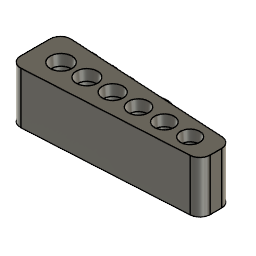
HoleDiaTest1.75mm_v3 (Autodesk Fusion 360 design; units mm, degrees)
Autodesk Fusion 360 part; units mm, degrees
sketch "Sketch1" plane through (0, 0, 0) normal (0, 0, 1) x (1, 0, 0)
  circle A0 centre (0, 0) radius 0.875
  circle A1 centre (2.5, 0) radius 0.85
  circle A2 centre (5, 0) radius 0.825
  circle A3 centre (-2.5, 0) radius 0.9
  circle A4 centre (-5, 0) radius 0.925
  circle A5 centre (-7.5, 0) radius 0.95
  line L0 (-7.5, 0) -> (5, 0) construction
  line L1 (5, 0) -> (7.5, 0) construction
  line L2 (-7.5, 0) -> (-10, 0) construction
  line L3 (-10, 2.5) -> (-10, -2.5)
  line L4 (7.5, 1.5) -> (7.5, -1.5)
  line L5 (7.5, 1.5) -> (-10, 2.5)
  line L6 (-10, -2.5) -> (7.5, -1.5)
  dimension "d1" = 1.75
  dimension "d2" = 1.7
  dimension "d3" = 1.65
  dimension "d4" = 1.8
  dimension "d5" = 1.85
  dimension "d6" = 1.9
  dimension "d7" = 2.5
  dimension "d8" = 2.5
  dimension "d9" = 2.5
  dimension "d10" = 2.5
  dimension "d11" = 2.5
  constraint coincident A5.centre L0.start
  constraint coincident A2.centre L0.end
  constraint horizontal L0
  constraint parallel L0 L1
  constraint parallel L0 L2
  constraint midpoint L2.end L3
  constraint perpendicular L2 L3
  constraint midpoint L1.end L4
  constraint perpendicular L1 L4
  measures "d1" diameter of A0
  measures "d2" diameter of A1
  measures "d3" diameter of A2
  measures "d4" diameter of A3
  measures "d5" diameter of A4
  measures "d6" diameter of A5
  measures "d7" distance of A4.centre A5.centre
  measures "d8" distance of A3.centre A4.centre
  measures "d9" distance of A0.centre A3.centre
  measures "d10" distance of A0.centre A1.centre
  measures "d11" distance of A1.centre A2.centre
extrude "Extrude1" add sketch "Sketch1" against normal blind 5
fillet "Fillet1" radius 1 4 edges at (7.5, 1.5, -2.5) (7.5, -1.5, -2.5) (-10, 2.5, -2.5) (-10, -2.5, -2.5)
chamfer "Chamfer1" distance 0.1 distance2 1 12 edges at (-8.3857, 0.3435, 0) (-5.8624, 0.3345, 0) (-3.3391, 0.3255, 0) (-0.8158, 0.3164, 0) (1.7075, 0.3074, 0) (4.2308, 0.2983, 0) (4.2308, -0.2983, -5) (1.7075, -0.3074, -5) (-0.8158, -0.3164, -5) (-3.3391, -0.3255, -5) (-5.8624, -0.3345, -5) (-8.3857, -0.3435, -5) measured on face at (-9.4833, 0, 0) measured on face at (-9.4833, 0, 0) measured on face at (-9.4833, 0, 0) measured on face at (-9.4833, 0, 0) measured on face at (-9.4833, 0, 0) measured on face at (-9.4833, 0, 0) measured on face at (-9.4833, 0, -5) measured on face at (-9.4833, 0, -5) measured on face at (-9.4833, 0, -5) measured on face at (-9.4833, 0, -5) measured on face at (-9.4833, 0, -5) measured on face at (-9.4833, 0, -5) tangent chain off
sketch "Sketch2" plane through (0.1098, 1.9223, 0) normal (0.05705, 0.998371, 0) x (-0.998371, 0.05705, 0)
  line L0 (9.0676, -5) -> (9.0676, 0)
  line L1 (9.0676, 0) -> (-6.4577, 0)
  line L2 (-6.4577, 0) -> (-6.4577, -5)
  line L3 (-6.4577, -5) -> (9.0676, -5)
  line L4 (8.5, -0.5) -> (-5, -0.5) construction
  line L5 (-5, -0.5) -> (-5, -4.5) construction
  line L6 (-5, -4.5) -> (8.5, -4.5) construction
  line L7 (8.5, -4.5) -> (8.5, -0.5) construction
  dimension "d22" = 4
  dimension "d23" = 0
  text T0 "1.75" font "Arial" height 4 align left top in box 13.5 x 4 at (8.5, -0.5) x (-1, 0) y (0, -1) spacing 1.01 kerned
extrude "Extrude2" add sketch "Sketch2" along normal blind 0.5 text T0
equation "d23 = '1.75'"
